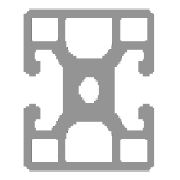
# Autodesk Inventor part: 10-240
Saved by Autodesk Inventor 2022 (Build 260153000, 153)
## iProperties
IsCustomPart: 1
Created: 2021-12-28
Part Number: 10-240
Material: Generico
Document SubType Name: Modeling
Designer: matte
Standards Organization: 40 series
Language: it-IT
Size Designation: 10-240
Categories: <MemberInstance><Categories><Category DisplayName="Forme strutturali" InternalName="089c4875-fa83-4c05-b084-43b9cc11f5ed" Mnemonic="GRDR"><CategoryParameter DisplayName="Massa per unità di lunghezza" InternalName="0bb95a10-148f-4027-a459-38d7b056702a" Mnemonic="shpmass"/><CategoryParameter DisplayName="Area sezione" InternalName="1ff91680-64b0-4202-b9a3-7fd3f94bba3b" Mnemonic="secarea"/><CategoryParameter DisplayName="Raggio di girazione (x)" InternalName="25778675-03e9-40c1-b6a8-4a9ed693320d" Mnemonic="gyrradx"/><CategoryParameter DisplayName="Modulo di rigidità torsionale" InternalName="26c1ec35-5026-4c63-ad0a-751cf684a536" Mnemonic="torrigmod"/><CategoryParameter DisplayName="Distanza del baricentro X-X" InternalName="26c9bdb8-9c79-4b4f-a92e-8e197583c9c4" Mnemonic="grcendistX"/><CategoryParameter DisplayName="ID membro precedente" InternalName="340afe4f-75d7-48d3-ab7d-943f3c3da468" Mnemonic="LegacyMemberID"/><CategoryParameter DisplayName="Lunghezza base" InternalName="42e34263-8f20-4d0e-ad48-bf1385b87c24" Mnemonic="shplen"/><CategoryParameter DisplayName="Momento di inerzia (y)" InternalName="4b9f58ea-bced-460e-81ea-3d29ca5a49e3" Mnemonic="inermomy"/><CategoryParameter DisplayName="Momento di inerzia (x)" InternalName="4cd780bc-73d7-43ac-917a-579e5cbd684d" Mnemonic="inermomx"/><CategoryParameter DisplayName="Punto di base personalizzato" InternalName="4f1d1b73-316d-484b-a3df-9cbabb16eb77" Mnemonic="shpBasePoint"/><CategoryParameter DisplayName="Altezza forma" InternalName="50274e7d-5ac0-4796-92cb-c59e54983c67" Mnemonic="shpheig"/><CategoryParameter DisplayName="Modulo sezione (y)" InternalName="59eaa5e9-d227-48dc-b6c1-6920f96e0f95" Mnemonic="secmody"/><CategoryParameter DisplayName="Designazione sezione" InternalName="5a64d034-428d-49c8-ba32-7619764de20f" Mnemonic="shpdes"/><CategoryParameter DisplayName="Modulo sezione (x)" InternalName="72cfad18-cf51-4ed4-aaa7-c6b224f8419f" Mnemonic="secmodx"/><CategoryParameter DisplayName="Modulo di sezione torsionale" InternalName="7c55a8dc-8844-49f9-a867-cc677b30ec9a" Mnemonic="torsecmod"/><CategoryParameter DisplayName="Larghezza forma" InternalName="7c717d54-a18f-4666-b4d4-573cce22c62c" Mnemonic="shpwdth"/><CategoryParameter DisplayName="Spessore seconda forma" InternalName="9251a8e1-85fd-4e47-af99-afdb762317d9" Mnemonic="shpthick2"/><CategoryParameter DisplayName="Guarnizione piatta creata" InternalName="9c666724-f362-4ea7-ac62-f6a007de5c69" Mnemonic="shpFGAuto"/><CategoryParameter DisplayName="Distanza del baricentro Y-Y" InternalName="bcc4fb17-7af4-436a-8f8c-d0aa3b0248c5" Mnemonic="grcendistY"/><CategoryParameter DisplayName="Raggio di girazione (y)" InternalName="bfa18ebe-1636-4dbe-8d42-b263e0b73184" Mnemonic="gyrrady"/><CategoryParameter DisplayName="Spessore forma" InternalName="d109cf76-8eb4-42fc-9800-4409734adc67" Mnemonic="shpthick"/><CategoryParameter DisplayName="Coefficiente di spostamento taglio" InternalName="de4c90c6-aaa8-468f-a335-6737b311b5d3" Mnemonic="shdispc"/><Category DisplayName="Altro" InternalName="f02205ff-2390-476f-921c-0b3185f88e84" Mnemonic="OTHSHP"><CategoryParameter DisplayName="Momento di inerzia (y)" InternalName="044c654e-f649-48ac-84cc-650a29ae31ca" Mnemonic="inermomy"/><CategoryParameter DisplayName="Spessore forma" InternalName="12b1a788-9233-48fd-a933-2df8ff42b15f" Mnemonic="shpthick"/><CategoryParameter DisplayName="Massa per unità di lunghezza" InternalName="2fd289d6-9394-4d2d-97e6-6659d7d4551d" Mnemonic="shpmass"/><CategoryParameter DisplayName="Raggio di girazione (y)" InternalName="743e1dfe-1bba-408b-b985-cf752b207386" Mnemonic="gyrrady"/><CategoryParameter DisplayName="Modulo sezione (y)" InternalName="88b8bff9-a616-4028-93d5-ed4f79680d13" Mnemonic="secmody"/><CategoryParameter DisplayName="Area sezione" InternalName="c46ecdf8-b6eb-4db9-8b25-30258930c1e3" Mnemonic="secarea"/><CategoryParameter DisplayName="Modulo sezione (x)" InternalName="cac70804-9d39-43bb-be17-56ea1f39a6c2" Mnemonic="secmodx"/><CategoryParameter DisplayName="Momento di inerzia (x)" InternalName="ec6737bc-264f-43ed-b0bd-f6d410c2718d" Mnemonic="inermomx"/><CategoryParameter DisplayName="Raggio di girazione (x)" InternalName="ee72c61e-565e-4fd6-b448-66e1e1abcb7e" Mnemonic="gyrradx"/></Category></Category><Category DisplayName="TipoDati" InternalName="23b78d0f-2648-40c6-8793-ca6db495c9e8" Mnemonic="DATATYPE"><CategoryParameter DisplayName="NomeVisualizzazione" InternalName="05415f3d-3907-474b-a020-eb9d644f4cf3" Mnemonic="DISPLAYNAME"/><CategoryParameter DisplayName="Norme" InternalName="0c0a119c-1e12-4c84-803f-101930972f5e" Mnemonic="STANDARD"/><CategoryParameter DisplayName="Descrizione" InternalName="13903e3d-64b1-4950-80da-f627842ea37f" Mnemonic="DESCRIPTION"/><CategoryParameter DisplayName="Designazione" InternalName="2675968c-4ce5-49e0-a4f5-552d29089031" Mnemonic="DESIGNATION"/><CategoryParameter DisplayName="Riga di default" InternalName="2af9ec52-faaa-4026-b378-f9fa4afca842" Mnemonic="DEFAULTROW"/><CategoryParameter DisplayName="Nome cartella" InternalName="3f06958e-8713-4116-9be7-ed6184ecc97b" Mnemonic="FOLDERNAME"/><CategoryParameter DisplayName="Guid revisione" InternalName="45a75005-10b1-4dfc-8d6d-dfe629f0b93c" Mnemonic="REVISIONGUID"/><CategoryParameter DisplayName="NomeFile" InternalName="8b46a4cc-9585-4fed-90c3-899f57e09a73" Mnemonic="FILENAME"/><CategoryParameter DisplayName="SocietàNorme" InternalName="8f5914e1-4693-403f-8ab5-d37768198c9d" Mnemonic="STDSORG"/><CategoryParameter DisplayName="Versione famiglia" InternalName="914462f6-6e19-4b14-ba84-155b9680b1d0" Mnemonic="FAMILYREVISION"/><CategoryParameter DisplayName="Revisione norme" InternalName="91d5a463-65c2-4fde-b823-3b7fea5e8e17" Mnemonic="STANDARDREVISION"/><CategoryParameter DisplayName="Revisione membro" InternalName="a65d44b9-392f-4f4f-857b-e4b3d54996fe" Mnemonic="MEMBERREVISION"/><CategoryParameter DisplayName="FormatoPianoRitaglio" InternalName="bc51e27b-3422-4e78-93ef-cec197ddf230" Mnemonic="CLIPFORMAT"/><CategoryParameter DisplayName="Produttore" InternalName="cd6c7a72-a28a-4e50-99a9-2c7f4e13e5ad" Mnemonic="MANUFACTURER"/><CategoryParameter DisplayName="NomeInterno" InternalName="cf1d0246-76d9-4b4a-8305-fa0409afb5c1" Mnemonic="INTERNALNAME"/><CategoryParameter DisplayName="Èmetrico" InternalName="e2385c5b-1ea4-4823-96a8-8de651266ec3" Mnemonic="ISMETRIC"/><Category DisplayName="Parte" InternalName="c0e0b642-3bcb-4cc8-9e80-f96d35c4afa4" Mnemonic="PART"><CategoryParameter DisplayName="Numero parte" InternalName="016b6077-bfbe-49bd-92c9-d8d59c39c941" Mnemonic="PARTNUMBER"/><CategoryParameter DisplayName="Numero di magazzino" InternalName="4dba7c1c-e26c-444e-836c-b08b433409a8" Mnemonic="STOCKNUMBER"/><CategoryParameter DisplayName="Chiave materiale" InternalName="5c9a8adb-dd2b-4535-b97f-0a94a95fe41f" Mnemonic="MATERIALKEY"/><CategoryParameter DisplayName="Materiale" InternalName="818a152a-d3c3-49ca-80ee-df7d91421b8e" Mnemonic="MATERIAL"/></Category></Category></Categories><FamilyTemplate Id="10-240"><FamilyTemplateParameters><FamilyTemplateParameter ObjectType="kModelParameterObject" ValueType="xs:double" Id="12" ObjectReferenceKey="d0"/><FamilyTemplateParameter ObjectType="kPartComponentDefinitionObject" ValueType="xs:string" Id="23" SubObjectId="Material"/><FamilyTemplateParameter ObjectType="kPropertyObject" ValueType="xs:string" Id="26" ObjectReferenceKey="{32853F0F-3444-11d1-9E93-0060B03C1CA6}" SubObjectId="5"/><FamilyTemplateParameter ObjectType="kPropertyObject" ValueType="xs:string" Id="27" ObjectReferenceKey="{32853F0F-3444-11d1-9E93-0060B03C1CA6}" SubObjectId="52"/></FamilyTemplateParameters></FamilyTemplate><CategoryParameterMap><ParamToTemplateMap><ParamToTemplate CategoryParameter="//CategoryParameter[@InternalName='cf1d0246-76d9-4b4a-8305-fa0409afb5c1']" ConstantValue="d6ff3bdf-0714-468a-95a3-b51ab3a761af"/><ParamToTemplate CategoryParameter="//CategoryParameter[@InternalName='45a75005-10b1-4dfc-8d6d-dfe629f0b93c']" ConstantValue="f65d2347-275f-4554-91ae-5ae26a1a182d"/><ParamToTemplate CategoryParameter="//CategoryParameter[@InternalName='3f06958e-8713-4116-9be7-ed6184ecc97b']" ConstantValue="10-240"/><ParamToTemplate CategoryParameter="//CategoryParameter[@InternalName='8f5914e1-4693-403f-8ab5-d37768198c9d']" ConstantValue="40 series"/><ParamToTemplate CategoryParameter="//CategoryParameter[@InternalName='0c0a119c-1e12-4c84-803f-101930972f5e']" TemplateParameter="18"/><ParamToTemplate CategoryParameter="//CategoryParameter[@InternalName='91d5a463-65c2-4fde-b823-3b7fea5e8e17']" TemplateParameter="19"/><ParamToTemplate CategoryParameter="//CategoryParameter[@InternalName='cd6c7a72-a28a-4e50-99a9-2c7f4e13e5ad']" TemplateParameter="20"/><ParamToTemplate CategoryParameter="//CategoryParameter[@InternalName='13903e3d-64b1-4950-80da-f627842ea37f']" TemplateParameter="22"/><ParamToTemplate CategoryParameter="//CategoryParameter[@InternalName='05415f3d-3907-474b-a020-eb9d644f4cf3']" ConstantValue="10-240"/><ParamToTemplate CategoryParameter="//CategoryParameter[@InternalName='914462f6-6e19-4b14-ba84-155b9680b1d0']" ConstantValue="11"/><ParamToTemplate CategoryParameter="//CategoryParameter[@InternalName='bc51e27b-3422-4e78-93ef-cec197ddf230']" ConstantValue="CF_INVENTOR.STDPARTS"/><ParamToTemplate CategoryParameter="//CategoryParameter[@InternalName='e2385c5b-1ea4-4823-96a8-8de651266ec3']" ConstantValue="true"/><ParamToTemplate CategoryParameter="//CategoryParameter[@InternalName='2af9ec52-faaa-4026-b378-f9fa4afca842']" ConstantValue="1"/><ParamToTemplate CategoryParameter="//CategoryParameter[@InternalName='9c666724-f362-4ea7-ac62-f6a007de5c69']" ConstantValue="1"/><ParamToTemplate CategoryParameter="//CategoryParameter[@InternalName='8b46a4cc-9585-4fed-90c3-899f57e09a73']" ConstantValue="10-240"/><ParamToTemplate CategoryParameter="//CategoryParameter[@InternalName='a65d44b9-392f-4f4f-857b-e4b3d54996fe']" ConstantValue="9fad4830-c198-42eb-8bed-0ea894f866c0"/><ParamToTemplate CategoryParameter="//CategoryParameter[@InternalName='a65d44b9-392f-4f4f-857b-e4b3d54996fe']" ConstantValue="9fad4830-c198-42eb-8bed-0ea894f866c0"/><ParamToTemplate CategoryParameter="//CategoryParameter[@InternalName='2675968c-4ce5-49e0-a4f5-552d29089031']" TemplateParameter="27"/><ParamToTemplate CategoryParameter="//CategoryParameter[@InternalName='818a152a-d3c3-49ca-80ee-df7d91421b8e']" TemplateParameter="23"/><ParamToTemplate CategoryParameter="//CategoryParameter[@InternalName='016b6077-bfbe-49bd-92c9-d8d59c39c941']" TemplateParameter="26"/><ParamToTemplate CategoryParameter="//CategoryParameter[@InternalName='42e34263-8f20-4d0e-ad48-bf1385b87c24']" TemplateParameter="12"/></ParamToTemplateMap></CategoryParameterMap></MemberInstance>
Density: 1 g/cm^3
Appearance: Default
MXEDIT: true
G_L: 4000,000 mm
Author: matte
Autodesk Inventor part; units mm, degrees
ref_plane "YZ Plane" through (0, 0, 0) normal (1, 0, 0) x (0, 1, 0)
ref_plane "Start Plane" through (0, 0, 0) normal (0, 1, 0) x (-1, 0, 0)
ref_plane "End Plane" through (0, 4000, 0) normal (0, 1, 0) x (-1, 0, 0)
sketch "Sketch1" plane through (0, 0, 0) normal (0, 1, 0) x (-1, 0, 0)
  line L0 (-7.6078, -17) -> (-7.6078, -12.74)
  arc A0 (-2.6078, -7.74) -> (-7.6078, -12.74) centre (-2.6078, -12.74) ccw
  line L1 (-2.6078, -7.74) -> (2.3922, -7.74)
  arc A1 (7.3922, -12.74) -> (2.3922, -7.74) centre (2.3922, -12.74) ccw
  line L2 (7.3922, -12.74) -> (7.3922, -17)
  arc A2 (6.1722, -18.22) -> (7.3922, -17) centre (6.1722, -17) ccw
  line L3 (6.1722, -18.22) -> (-6.3878, -18.22)
  arc A3 (-7.6078, -17) -> (-6.3878, -18.22) centre (-6.3878, -17) ccw
  line L4 (9.1722, -17) -> (9.1722, -13)
  arc A4 (10.3922, -11.78) -> (9.1722, -13) centre (10.3922, -13) ccw
  line L5 (10.3922, -11.78) -> (17, -11.78)
  arc A5 (18.22, -13) -> (17, -11.78) centre (17, -13) ccw
  line L6 (18.22, -13) -> (18.22, -17)
  arc A6 (17, -18.22) -> (18.22, -17) centre (17, -17) ccw
  line L7 (17, -18.22) -> (10.3922, -18.22)
  arc A7 (9.1722, -17) -> (10.3922, -18.22) centre (10.3922, -17) ccw
  line L8 (-18.22, 13) -> (-18.22, 17)
  arc A8 (-17, 18.22) -> (-18.22, 17) centre (-17, 17) ccw
  line L9 (-17, 18.22) -> (-10.6078, 18.22)
  arc A9 (-9.3878, 17) -> (-10.6078, 18.22) centre (-10.6078, 17) ccw
  line L10 (-9.3878, 17) -> (-9.3878, 13)
  arc A10 (-10.6078, 11.78) -> (-9.3878, 13) centre (-10.6078, 13) ccw
  line L11 (-10.6078, 11.78) -> (-17, 11.78)
  arc A11 (-18.22, 13) -> (-17, 11.78) centre (-17, 13) ccw
  line L12 (9.1722, 13) -> (9.1722, 17)
  arc A12 (10.3922, 18.22) -> (9.1722, 17) centre (10.3922, 17) ccw
  line L13 (10.3922, 18.22) -> (17, 18.22)
  arc A13 (18.22, 17) -> (17, 18.22) centre (17, 17) ccw
  line L14 (18.22, 17) -> (18.22, 13)
  arc A14 (17, 11.78) -> (18.22, 13) centre (17, 13) ccw
  line L15 (17, 11.78) -> (10.3922, 11.78)
  arc A15 (9.1722, 13) -> (10.3922, 11.78) centre (10.3922, 13) ccw
  line L16 (-18.22, -17) -> (-18.22, -13)
  arc A16 (-17, -11.78) -> (-18.22, -13) centre (-17, -13) ccw
  line L17 (-17, -11.78) -> (-10.6078, -11.78)
  arc A17 (-9.3878, -13) -> (-10.6078, -11.78) centre (-10.6078, -13) ccw
  line L18 (-9.3878, -13) -> (-9.3878, -17)
  arc A18 (-10.6078, -18.22) -> (-9.3878, -17) centre (-10.6078, -17) ccw
  line L19 (-10.6078, -18.22) -> (-17, -18.22)
  arc A19 (-18.22, -17) -> (-17, -18.22) centre (-17, -17) ccw
  line L20 (-7.6078, 12.74) -> (-7.6078, 17)
  arc A20 (-6.3878, 18.22) -> (-7.6078, 17) centre (-6.3878, 17) ccw
  line L21 (-6.3878, 18.22) -> (6.1722, 18.22)
  arc A21 (7.3922, 17) -> (6.1722, 18.22) centre (6.1722, 17) ccw
  line L22 (7.3922, 17) -> (7.3922, 12.74)
  arc A22 (2.3922, 7.74) -> (7.3922, 12.74) centre (2.3922, 12.74) ccw
  line L23 (2.3922, 7.74) -> (-2.6078, 7.74)
  arc A23 (-7.6078, 12.74) -> (-2.6078, 7.74) centre (-2.6078, 12.74) ccw
  arc A24 (-16, -7) -> (-15.5, -6.5) centre (-16, -6.5) ccw
  line L24 (-15.5, -6.5) -> (-15.5, -5)
  arc A25 (-15.5, -5) -> (-16.5, -4) centre (-16.5, -5) ccw
  line L25 (-16.5, -4) -> (-18.3248, -4)
  line L26 (-20, -16) -> (-20, -17)
  arc A26 (-20, -17) -> (-17, -20) centre (-17, -17) ccw
  line L27 (-17, -20) -> (17, -20)
  line L28 (20, -17) -> (20, -16)
  line L29 (18.5, -4) -> (16.5, -4)
  line L30 (-17, -9) -> (-17, -8)
  arc A27 (20, -5.5) -> (18.5, -4) centre (18.5, -5.5) ccw
  arc A28 (16.5, -4) -> (15.5, -5) centre (16.5, -5) ccw
  line L31 (15.5, -5) -> (15.5, -6.5)
  arc A29 (15.5, -6.5) -> (16, -7) centre (16, -6.5) ccw
  arc A30 (17, -8) -> (16, -7) centre (16, -8) ccw
  line L32 (17, -8) -> (17, -9)
  arc A31 (16, -10) -> (17, -9) centre (16, -9) ccw
  line L33 (16, -10) -> (12.3321, -10)
  arc A32 (11.9786, -9.8536) -> (12.3321, -10) centre (12.3321, -9.5) ccw
  line L34 (11.9786, -9.8536) -> (7.8964, -5.7714)
  arc A33 (7.75, -5.4179) -> (7.8964, -5.7714) centre (8.25, -5.4179) ccw
  line L35 (7.75, -5.4179) -> (7.75, 5.4179)
  arc A34 (7.8964, 5.7714) -> (7.75, 5.4179) centre (8.25, 5.4179) ccw
  line L36 (7.8964, 5.7714) -> (11.9786, 9.8536)
  arc A35 (12.3321, 10) -> (11.9786, 9.8536) centre (12.3321, 9.5) ccw
  line L37 (12.3321, 10) -> (16, 10)
  arc A36 (17, 9) -> (16, 10) centre (16, 9) ccw
  line L38 (17, 9) -> (17, 8)
  arc A37 (16, 7) -> (17, 8) centre (16, 8) ccw
  arc A38 (16, 7) -> (15.5, 6.5) centre (16, 6.5) ccw
  line L39 (15.5, 6.5) -> (15.5, 5)
  arc A39 (15.5, 5) -> (16.5, 4) centre (16.5, 5) ccw
  line L40 (16.5, 4) -> (18.3248, 4)
  line L41 (20, 16) -> (20, 17)
  line L42 (17, 20) -> (-17, 20)
  arc A40 (-17, 20) -> (-20, 17) centre (-17, 17) ccw
  line L43 (-20, 17) -> (-20, 16)
  line L44 (-18.5, 4) -> (-16.5, 4)
  arc A41 (-20, 5.5) -> (-18.5, 4) centre (-18.5, 5.5) ccw
  arc A42 (-16.5, 4) -> (-15.5, 5) centre (-16.5, 5) ccw
  line L45 (-15.5, 5) -> (-15.5, 6.5)
  arc A43 (-15.5, 6.5) -> (-16, 7) centre (-16, 6.5) ccw
  arc A44 (-17, 8) -> (-16, 7) centre (-16, 8) ccw
  line L46 (-17, 8) -> (-17, 9)
  arc A45 (-16, 10) -> (-17, 9) centre (-16, 9) ccw
  line L47 (-16, 10) -> (-12.3321, 10)
  arc A46 (-11.9786, 9.8536) -> (-12.3321, 10) centre (-12.3321, 9.5) ccw
  line L48 (-11.9786, 9.8536) -> (-7.8964, 5.7714)
  arc A47 (-7.75, 5.4179) -> (-7.8964, 5.7714) centre (-8.25, 5.4179) ccw
  line L49 (-7.75, 5.4179) -> (-7.75, -5.4179)
  arc A48 (-7.8964, -5.7714) -> (-7.75, -5.4179) centre (-8.25, -5.4179) ccw
  line L50 (-7.8964, -5.7714) -> (-11.9786, -9.8536)
  arc A49 (-12.3321, -10) -> (-11.9786, -9.8536) centre (-12.3321, -9.5) ccw
  line L51 (-12.3321, -10) -> (-16, -10)
  arc A50 (-17, -9) -> (-16, -10) centre (-16, -9) ccw
  arc A51 (-16, -7) -> (-17, -8) centre (-16, -8) ccw
  circle A52 centre (0, 0) radius 3.35
  line L52 (-20, 17) -> (-20, 5.5)
  line L53 (20, 17) -> (20, 5.5)
  arc A53 (18.5, 4) -> (20, 5.5) centre (18.5, 5.5) ccw
  arc A54 (20, 17) -> (17, 20) centre (17, 17) ccw
  line L54 (18.3248, 4) -> (18.5, 4)
  line L55 (20, -5.5) -> (20, -17)
  arc A55 (17, -20) -> (20, -17) centre (17, -17) ccw
  line L56 (-20, -5.5) -> (-20, -17)
  line L57 (-18.3248, -4) -> (-18.5, -4)
  arc A56 (-18.5, -4) -> (-20, -5.5) centre (-18.5, -5.5) ccw
  constraints: 116 end point, 112 point on circle, 57 centre point, 30 vertical, 24 horizontal, 4 point on line, 233 other
extrude "Body" add sketch "Sketch1" along normal up to surface (4000 mm away) from surface at 0
sketch "Sketch2" plane through (0, 0, 0) normal (0, 1, 0) x (-1, 0, 0)
  line L0 (0, 0) -> (10, 0)
ref_plane "Work Plane3" through (0, 0, 0) normal (0, 0, -1) x (-1, 0, 0)
sketch "Sketch3" plane through (0, 0, 0) normal (0, 0, -1) x (-1, 0, 0)
  line L0 (-2, 0) -> (12, 0)
  line L1 (-2, 4000) -> (12, 4000)
  dimension "d7" = 4000
  measures "d7" distance between parallel lines of L0 L1
equation "\"G_OFFSET_START\" = 0"
equation "\"G_OFFSET_END\" = 0"
equation "\"G_L\" = d7"
body "Solid1"
